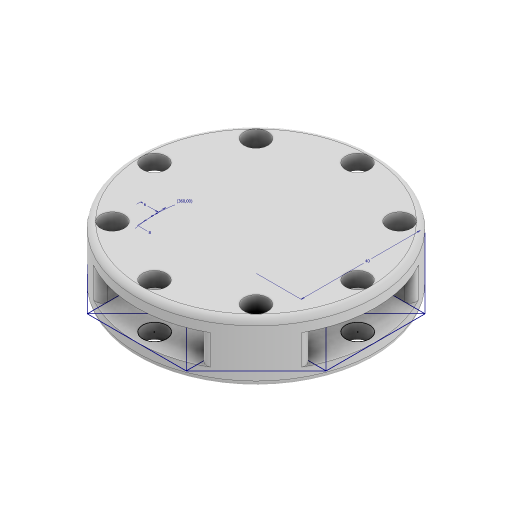
# Autodesk Inventor part: riemschijf
Saved by Autodesk Inventor 2024.2 (Build 282272000, 272)
## iProperties
Created: 2024-11-11
Part Number: riemschijf
Material: Generic
Document SubType Name: Modeling
Designer: Bram
Density: 1 g/cm^3
Appearance: Default
Author: Bram
Autodesk Inventor part; units mm, degrees
ref_plane "YZ Plane" through (0, 0, 0) normal (1, 0, 0) x (0, 1, 0)
ref_plane "XZ Plane" through (0, 0, 0) normal (0, 1, 0) x (-1, 0, 0)
ref_plane "XY Plane" through (0, 0, 0) normal (0, 0, 1) x (1, 0, 0)
sketch "Sketch1" plane through (0, 0, 0) normal (0, 1, 0) x (-1, 0, 0)
  line L0 (40, -16.5685) -> (16.5685, -40)
  line L1 (16.5685, -40) -> (-16.5685, -40)
  line L2 (-16.5685, -40) -> (-40, -16.5685)
  line L3 (-40, -16.5685) -> (-40, 16.5685)
  line L4 (-40, 16.5685) -> (-16.5685, 40)
  line L5 (-16.5685, 40) -> (16.5685, 40)
  line L6 (16.5685, 40) -> (40, 16.5685)
  line L7 (40, 16.5685) -> (40, -16.5685)
  line L8 (0, 0) -> (6.1053, 0)
  line L9 (16.5685, 40) -> (-40, -16.5685)
  line L10 (40, 16.5685) -> (-16.5685, -40)
  line L11 (40, -16.5685) -> (-40, -16.5685)
  line L12 (40, 16.5685) -> (-40, 16.5685)
  line L13 (-16.5685, 40) -> (-16.5685, -40)
  line L14 (16.5685, 40) -> (16.5685, -40)
  line L15 (16.5685, -40) -> (-40, 16.5685)
  line L16 (-16.5685, 40) -> (40, -16.5685)
  circle A0 centre (34, 0) radius 4
  circle A1 centre (24.0416, 24.0416) radius 4
  circle A2 centre (0, 34) radius 4
  circle A3 centre (-24.0416, 24.0416) radius 4
  circle A4 centre (-34, 0) radius 4
  circle A5 centre (-24.0416, -24.0416) radius 4
  circle A6 centre (0, -34) radius 4
  circle A7 centre (24.0416, -24.0416) radius 4
  point P0 (40, 0)
  point P1 (-16.5685, -16.5685)
  point P2 (16.5685, -40)
  point P3 (16.5685, -16.5685)
  point P4 (-16.5685, 16.5685)
  point P5 (16.5685, 16.5685)
  dimension "d0" = 8
  dimension "d1" = 40
  dimension "d2" = 6
  dimension "d5" = 360
  constraints: 34 end point, 8 centre point, 3 horizontal, 3 parallel, 3 perpendicular, 1 coincident, 1 midpoint, 1 vertical, 34 other
  measures "d0" diameter of A0
  measures "d1" distance from line of point (0, 0) L1
  measures "d2" distance of point (40, 0) A0.centre
extrude "Extrusion1" add sketch "Sketch1" along normal blind 10 contours L0 L14 L11 | L12 L14 L6 | L2 L11 L13 | L13 L12 L4
extrude "Extrusion2" add sketch "Sketch1" against normal blind 5
fillet "Fillet1" radius 40 8 edges at (40, -2.5, 16.5685) (40, -2.5, -16.5685) (16.5685, -2.5, -40) (-16.5685, -2.5, -40) (-40, -2.5, -16.5685) (-40, -2.5, 16.5685) (-16.5685, -2.5, 40) (16.5685, -2.5, 40)
sketch "Sketch2" plane through (0, 10, 0) normal (0, 1, 0) x (1, 0, 0)
  circle A0 centre (0, 0) radius 40
  circle A1 centre (24.0416, -24.0416) radius 4 projected
  arc A2 (16.5685, -36.4072) -> (36.4072, -16.5685) centre (0, 0) ccw projected
  line L0 (16.5685, -36.4072) -> (16.5685, -16.5685) projected
  line L1 (16.5685, -16.5685) -> (36.4072, -16.5685) projected
  arc A3 (-36.4072, -16.5685) -> (-16.5685, -36.4072) centre (0, 0) ccw projected
  line L2 (-36.4072, -16.5685) -> (-16.5685, -16.5685) projected
  line L3 (-16.5685, -16.5685) -> (-16.5685, -36.4072) projected
  circle A4 centre (-24.0416, -24.0416) radius 4 projected
  arc A5 (-16.5685, 36.4072) -> (-36.4072, 16.5685) centre (0, 0) ccw projected
  line L4 (-16.5685, 36.4072) -> (-16.5685, 16.5685) projected
  line L5 (-16.5685, 16.5685) -> (-36.4072, 16.5685) projected
  circle A6 centre (-24.0416, 24.0416) radius 4 projected
  circle A7 centre (24.0416, 24.0416) radius 4 projected
  arc A8 (36.4072, 16.5685) -> (16.5685, 36.4072) centre (0, 0) ccw projected
  line L6 (36.4072, 16.5685) -> (16.5685, 16.5685) projected
  line L7 (16.5685, 16.5685) -> (16.5685, 36.4072) projected
  circle A9 centre (0, 34) radius 4 projected
  circle A10 centre (0, -34) radius 4 projected
  circle A11 centre (34, 0) radius 4 projected
  circle A12 centre (-34, 0) radius 4 projected
  constraints: 1 coincident, 2 other
extrude "Extrusion3" add sketch "Sketch2" along normal blind 5
fillet "Fillet2" radius 2 9 edges at (-40, 15, 0) (15.3073, -5, 36.9552) (-15.3073, -5, 36.9552) (36.9552, -5, 15.3073) (36.9552, -5, -15.3073) (15.3073, -5, -36.9552) (-15.3073, -5, -36.9552) (-36.9552, -5, -15.3073) (-36.9552, -5, 15.3073)
fillet "Fillet3" radius 2 12 edges at (-36.4072, 5, 16.5685) (-16.5685, 5, 36.4072) (-36.4072, 5, -16.5685) (-16.5685, 5, -16.5685) (-16.5685, 5, -36.4072) (-16.5685, 5, 16.5685) (16.5685, 5, 36.4072) (16.5685, 5, 16.5685) (16.5685, 5, -16.5685) (16.5685, 5, -36.4072) (36.4072, 5, -16.5685) (36.4072, 5, 16.5685)
body "Solid1"
